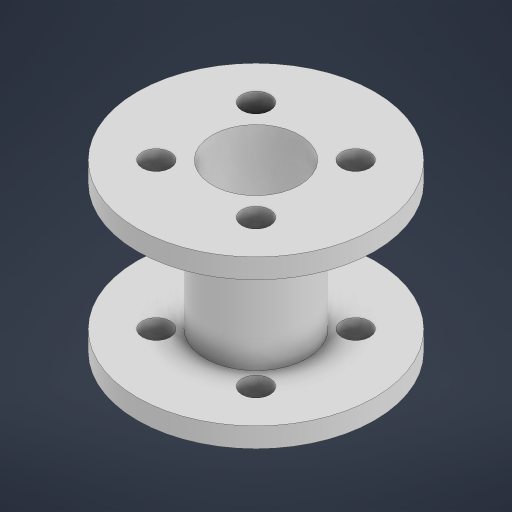
# Autodesk Inventor part: Slide_Climb_Spool
Saved by Autodesk Inventor 2023 (Build 270158000, 158)
## iProperties
Created: 2024-02-27
Part Number: Slide_Climb_Spool
Material: Generic
Document SubType Name: Modeling
Designer: kelle
Density: 1 g/cm^3
Appearance: Default
Author: kelle
Autodesk Inventor part; units mm, degrees
ref_plane "YZ Plane" through (0, 0, 0) normal (1, 0, 0) x (0, 1, 0)
ref_plane "XZ Plane" through (0, 0, 0) normal (0, 1, 0) x (-1, 0, 0)
ref_plane "XY Plane" through (0, 0, 0) normal (0, 0, 1) x (1, 0, 0)
sketch "Sketch1" plane through (0, 0, 0) normal (0, 0, 1) x (1, 0, 0)
  line L0 (-5, -10.16) -> (5, -10.16)
  line L1 (5, -10.16) -> (5, 10.16)
  line L2 (5, 10.16) -> (-5, 10.16)
  line L3 (-5, 10.16) -> (-5, -10.16)
  line L4 (-5, -10.16) -> (5, 10.16) construction
  line L5 (5, -10.16) -> (-5, 10.16) construction
  line L6 (5, 10.16) -> (8.1852, 10.16)
  line L7 (8.1852, 10.16) -> (8.1852, -10.16)
  line L8 (8.1852, -10.16) -> (5, -10.16)
  line L9 (5, -10.16) -> (5, 10.16)
  line L10 (0, 10.16) -> (0, -10.16)
  line L11 (0, 10.16) -> (19.05, 10.16)
  line L12 (19.05, 10.16) -> (19.05, 13.335)
  line L13 (19.05, 13.335) -> (0, 13.335)
  line L14 (0, 13.335) -> (0, 10.16)
  line L15 (0, -10.16) -> (19.05, -10.16)
  line L16 (19.05, -10.16) -> (19.05, -13.335)
  line L17 (19.05, -13.335) -> (0, -13.335)
  line L18 (0, -13.335) -> (0, -10.16)
  point P0 (0, 0)
  point P1 (8.1852, -10.16)
  dimension "d0" = 10
  dimension "d1" = 20.32
  dimension "d2" = 3.1852
  dimension "d3" = 19.05
  dimension "d4" = 3.175
  dimension "d5" = 19.05
  dimension "d6" = 3.175
  constraints: 38 end point, 8 parallel, 4 horizontal, 4 midpoint, 4 perpendicular
  measures "d0" distance of L2.end L1.end
  measures "d1" distance of L1.end L0.end
  measures "d2" distance of L7.end L8.end
  measures "d3" distance of L13.end L12.end
  measures "d4" distance of L12.end L11.end
  measures "d5" distance of L16.end L17.end
  measures "d6" distance of L15.end L16.end
revolve "Revolution1" add sketch "Sketch1" angle 360 about axis through (0, 10.16, 0) along (0, -1, 0) contours L0 L8 L15 L16 L17 L18 | L1 L6 L7 L8 | L14 L13 L12 L11 L6 L2
sketch "Sketch2" plane through (0, 13.335, 0) normal (0, 1, 0) x (1, 0, 0)
  circle A0 centre (0, 0) radius 7
  line L0 (8, -8) -> (-8, -8)
  line L1 (-8, -8) -> (-8, 8)
  line L2 (-8, 8) -> (8, 8)
  line L3 (8, 8) -> (8, -8)
  line L4 (8, -8) -> (-8, 8) construction
  line L5 (-8, -8) -> (8, 8) construction
  circle A1 centre (-8, 8) radius 2.25
  circle A2 centre (8, 8) radius 2.25
  circle A3 centre (8, -8) radius 2.25
  circle A4 centre (-8, -8) radius 2.25
  dimension "d8" = 14
  dimension "d11" = 16
  dimension "d12" = 16
  dimension "d13" = 4.5
  dimension "d14" = 4.5
  dimension "d15" = 4.5
  dimension "d16" = 4.5
  constraints: 12 end point, 5 centre point, 5 coincident, 2 midpoint, 2 parallel, 1 horizontal, 1 perpendicular
  measures "d8" diameter of A0
  measures "d11" distance of L1.end L2.end
  measures "d12" distance of L0.end L1.end
  measures "d13" diameter of A1
  measures "d14" diameter of A2
  measures "d15" diameter of A3
  measures "d16" diameter of A4
extrude "Extrusion1" cut sketch "Sketch2" against normal through all contours A0 | A4 L1 L0 | L0 L1 A4 | A3 L3 L0 | L0 L3 A3 | A1 L2 L1 | L1 L2 A1 | A2 L2 L3 | L3 L2 A2
body "Solid1"
